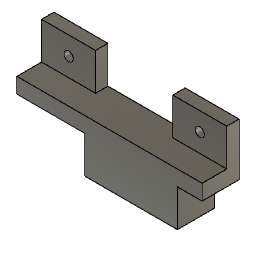
Fixation Tableau (Autodesk Fusion 360 design; units mm, degrees)
Autodesk Fusion 360 part; units mm, degrees
note: some values were not read from the file. Set by a fixed rule: which sketch regions a step uses.
sketch "Esquisse1" plane through (0, 0, 0) normal (0, 0, 1) x (1, 0, 0)
  line L0 (30, 4) -> (-30, 4)
  line L1 (-30, 4) -> (-30, -4)
  line L2 (-30, -4) -> (30, -4)
  line L3 (30, -4) -> (30, 4)
  line L4 (30, 4) -> (-30, -4) construction
  line L5 (-30, 4) -> (30, -4) construction
  dimension "d1" = 60
  dimension "d2" = 8
  constraint horizontal L0
  constraint perpendicular L0 L1
  constraint parallel L0 L2
  constraint parallel L1 L3
  constraint coincident L4 origin
  constraint coincident L5 origin
  measures "d1" distance of L1.end L2.end
  measures "d2" distance of L0.end L1.end
extrude "Extrusion1" add sketch "Esquisse1" along normal blind 5 makes body 1
sketch "Esquisse2" plane through (0, 0, 5) normal (0, 0, 1) x (-1, 0, 0)
  line L0 (-30, 4) -> (-30, -4)
  line L1 (-30, -4) -> (30, -4)
  line L2 (30, -4) -> (30, 4)
  line L3 (30, 4) -> (-30, 4)
  line L4 (8, 4) -> (-22, 4)
  line L5 (-22, 4) -> (-22, -8)
  line L6 (-22, -8) -> (8, -8)
  line L7 (8, -8) -> (8, 4)
  line L8 (0, 12.5546) -> (0, -11.3614) construction
  line L9 (8, -2) -> (-22, -2) construction
  circle A0 centre (0, -2) radius 4
  circle A1 centre (-15, -2) radius 4
  line L10 (8, 4) -> (-22, 4)
  line L11 (0, 2) -> (-15, 2)
  line L12 (0, -6) -> (-15, -6)
  dimension "d5" = 30
  dimension "d6" = 8
  dimension "d7" = 12
  dimension "d11" = 8
  dimension "d12" = 8
  dimension "d13" = 7
  constraint horizontal L4
  constraint vertical L5
  constraint horizontal L6
  constraint vertical L7
  constraint coincident L3 L4.start
  constraint perpendicular L6 L8
  constraint vertical origin L8.end
  constraint midpoint L7 L9.start
  constraint midpoint L5 L9.end
  constraint coincident L9 A0.centre
  constraint coincident L8 A0.centre
  constraint coincident L9 A1.centre
  constraint coincident A0 L11.start
  constraint coincident L8 L11.start
  constraint coincident A1 L11.end
  constraint tangent A1 L11
  constraint coincident A0 L12.start
  constraint coincident L8 L12.start
  constraint coincident A1 L12.end
  constraint tangent A1 L12
  measures "d5" distance of L5.end L6.end
  measures "d6" distance of L7 L8
  measures "d7" distance of L4 L6
  measures "d11" diameter of A0
  measures "d12" diameter of A1
  measures "d13" distance of L5 A1.centre
extrude "Extrusion2" add sketch "Esquisse2" against normal blind 15 separate body contours L1 L3 L4 L5 L7 A0 A1 L10 L11 | L1 L5 L6 L7 A0 A1 L12 makes body 2
sketch "Esquisse3" plane through (0, 0, -10) normal (0, 0, -1) x (1, 0, 0)
  line L0 (0, 2) -> (15, 2)
  arc A0 (15, -6) -> (15, 2) centre (15, -2) ccw
  line L1 (15, -6) -> (0, -6)
  arc A1 (0, 2) -> (0, -6) centre (0, -2) ccw
  line L2 (22, 4) -> (-8, 4)
  line L3 (-8, 4) -> (-8, -8)
  line L4 (-8, -8) -> (22, -8)
  line L5 (22, -8) -> (22, 4)
  circle A2 centre (0, -2) radius 2
  circle A3 centre (15, -2) radius 4
  line L6 (0, 0) -> (11.5359, 0)
  line L7 (0, -4) -> (11.5359, -4)
  dimension "d16" = 4
  dimension "d17" = 8
  constraint concentric A1 A2
  constraint concentric A0 A3
  constraint coincident A2 L6.start
  constraint coincident A3 L6.end
  constraint tangent A2 L6
  constraint parallel L0 L6
  constraint coincident A2 L7.start
  constraint coincident A3 L7.end
  constraint tangent A2 L7
  constraint parallel L6 L7
  measures "d16" diameter of A2
  measures "d17" diameter of A3
extrude "Extrusion3" add sketch "Esquisse3" along normal blind 2 contours L0 L1 A1 A2 A3 L6 L7 | L2 L3 L4 L5 bodies 2
sketch "Esquisse4" plane through (0, 4, 0) normal (0, 1, 0) x (-1, 0, 0)
  line L0 (-30, 0) -> (30, 0)
  line L1 (30, 0) -> (30, 5)
  line L2 (30, 5) -> (-30, 5)
  line L3 (-30, 5) -> (-30, 0)
  line L4 (15, 10.1786) -> (15, -11.9176) construction
  line L5 (0, 1.75) -> (0, 22.5) construction
  line L6 (-30, 0) -> (-12.5, 0)
  line L7 (-12.5, 0) -> (-12.5, 17)
  line L8 (-12.5, 17) -> (-30, 17)
  line L9 (-30, 17) -> (-30, 0)
  line L10 (30, 0) -> (12.5, 0)
  line L11 (12.5, 0) -> (12.5, 17)
  line L12 (12.5, 17) -> (30, 17)
  line L13 (30, 17) -> (30, 0)
  dimension "d21" = 17
  dimension "d22" = 17
  dimension "d38" = 25
  constraint perpendicular L2 L4
  constraint horizontal L6
  constraint vertical L7
  constraint horizontal L8
  constraint vertical L9
  constraint coincident L0.start L3.end
  constraint horizontal L10
  constraint vertical L11
  constraint horizontal L12
  constraint vertical L13
  constraint coincident L0.end L1.start
  measures "d21" distance of L0.start L8.end
  measures "d22" distance of L0.end L12.end
  measures "d38" distance of L7.end L11.end
extrude "Extrusion4" add sketch "Esquisse4" along normal blind 4 contours L0 L2 L3 L6 L7 L9 | L2 L7 L8 L9 | L0 L1 L2 L10 L11 L13 | L2 L11 L12 L13 bodies 2 1
sketch "Esquisse5" plane through (0, 0, 5) normal (0, 0, 1) x (-1, 0, 0)
  arc A0 (0, -6) -> (3.4641, -4) centre (0, -2) ccw
  line L0 (0, -6) -> (-12.5, -6)
  line L1 (-12.5, -8) -> (8, -8)
  line L2 (8, -8) -> (8, -4)
  line L3 (8, -4) -> (12.5, -4)
  line L4 (12.5, -4) -> (30, -4)
  line L5 (30, -4) -> (30, 4)
  line L6 (30, 4) -> (-30, 4)
  line L7 (-30, 4) -> (-30, -4)
  line L8 (-30, -4) -> (-12.5, -4)
  line L9 (-12.5, -4) -> (3.4641, -4)
  line L10 (8, -8) -> (-22, -8)
  line L11 (-22, -8) -> (-22, -4)
  line L12 (-22, -4) -> (8, -4)
  line L13 (8, -4) -> (8, -8)
  line L14 (-12.5, -6) -> (-12.5, -8)
  point P0 (-22, 4)
  constraint horizontal L10
  constraint vertical L11
  constraint horizontal L12
  constraint vertical L13
  constraint coincident L8 L11.end
  constraint coincident L1.end L2.start
  constraint vertical L11.end P0
extrude "Extrusion5" add sketch "Esquisse5" against normal blind 5 contours A0 L0 L8 L9 L10 L11 L12 L14 | A0 L0 L1 L2 L10 L12 L13 L14 bodies 2
sketch "Esquisse6" plane through (0, 8, 0) normal (0, 1, 0) x (-1, 0, 0)
  line L0 (30, 17) -> (12.5, 17)
  line L1 (12.5, 17) -> (12.5, 0)
  line L2 (12.5, 0) -> (30, 0)
  line L3 (30, 0) -> (30, 17)
  line L4 (30, 17) -> (12.5, 5) construction
  line L5 (12.5, 17) -> (30, 5) construction
  point P0 (21.25, 11)
  point P1 (12.5, 5)
  constraint coincident L0.start L3.end
  constraint coincident L1 P1
  constraint coincident L0.end L1.start
  constraint coincident L3 L5.end
  constraint midpoint P0 L4
  constraint horizontal L5.end P1
  constraint coincident P1 L4.end
hole "Perçage1" at (-21.25, 8, 11) direction (0, -1, 0) diameter 3 end through all countersink diameter 6 countersink angle 90 bodies 2
sketch "Esquisse8" plane through (0, 8, 0) normal (0, 1, 0) x (-1, 0, 0)
  line L0 (12.5, 0) -> (30, 0)
  line L1 (-30, 17) -> (-12.5, 5) construction
  line L2 (-12.5, 17) -> (-30, 5) construction
  circle A0 centre (21.25, 11) radius 3
  line L3 (30, 17) -> (12.5, 17)
  line L4 (12.5, 17) -> (12.5, 0)
  line L5 (30, 0) -> (30, 17)
  point P0 (-21.25, 11)
  constraint horizontal L1.end L2.end
  constraint midpoint P0 L2
hole "Perçage2" at (21.25, 8, 11) direction (0, -1, 0) diameter 3 end through all countersink diameter 6 countersink angle 90 bodies 2
sketch "Esquisse9" plane through (-12.5, 0, 0) normal (1, 0, 0) x (0, 1, 0)
  line L0 (4, 5) -> (4, 0)
  line L1 (4, 0) -> (8, 0)
  line L2 (8, 0) -> (8, 17)
  line L3 (8, 17) -> (4, 17)
  line L4 (4, 17) -> (4, 5)
  line L5 (8, 0) -> (4, 0)
  line L6 (4, 0) -> (4, 5)
  line L7 (4, 5) -> (8, 5)
  line L8 (8, 5) -> (8, 0)
  constraint horizontal L5
  constraint vertical L6
  constraint horizontal L7
  constraint vertical L8
  constraint coincident L0.start L4.end
  constraint coincident L1.end L2.start
extrude "Extrusion6" add sketch "Esquisse9" along normal up to surface (4.5 mm away) contours L0 L1 L2 L5 L6 L7 L8 bodies 2
